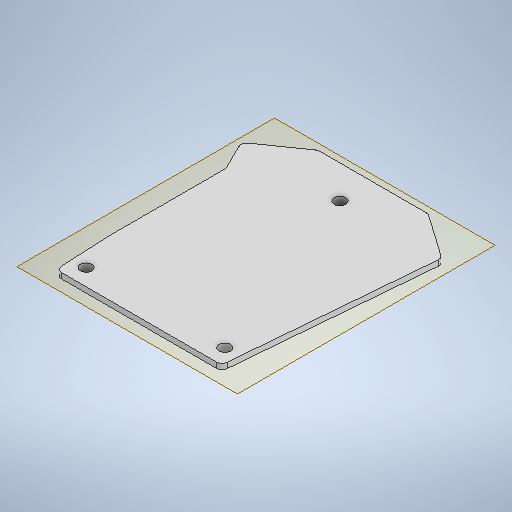
# Autodesk Inventor part: Deckel_oberteil
Saved by Autodesk Inventor 2025.1 (Build 291241000, 241)
## iProperties
Created: 2025-02-01
Part Number: Deckel_oberteil
Material: Generisch
Document SubType Name: Modeling
Designer: joebe
Density: 1 g/cm^3
Appearance: Vorgabe
Author: joebe
Autodesk Inventor part; units mm, degrees
ref_plane "YZ Plane" through (0, 0, 0) normal (1, 0, 0) x (0, 1, 0)
ref_plane "XZ Plane" through (0, 0, 0) normal (0, 1, 0) x (-1, 0, 0)
ref_plane "XY Plane" through (0, 0, 0) normal (0, 0, 1) x (1, 0, 0)
ref_plane "Arbeitsebene1" through (0, 0, 0) normal (0, 0, 1) x (1, 0, 0)
sketch "Skizze1" plane through (0, 0, 0) normal (0, 0, 1) x (1, 0, 0)
  line L0 (-29, -22.45) -> (-29, 20.1) projected
  line L1 (-29.2058, 20.9837) -> (-32.4027, 27.4738) projected
  line L2 (-17.2708, 40.1383) -> (-31.7557, 29.9959) projected
  line L3 (-16.1236, 40.5) -> (16.1236, 40.5) projected
  line L4 (33.1958, 28.9875) -> (17.2708, 40.1383) projected
  line L5 (34.0411, 27.1762) -> (28.1661, -40.5) projected
  line L6 (28.1661, -40.5) -> (-28.0975, -40.5) projected
  line L7 (-28.0975, -40.5) -> (-29, -22.45) projected
  line L8 (-30.9975, -22.5499) -> (-30.095, -40.5999) projected
  line L9 (-28.0975, -42.5) -> (28.1661, -42.5) projected
  line L10 (30.1586, -40.673) -> (36.2833, 29.879) projected
  line L11 (35.4379, 31.6903) -> (20.5166, 42.1383) projected
  line L12 (19.3694, 42.5) -> (-19.3694, 42.5) projected
  line L13 (-20.5166, 42.1383) -> (-34.9783, 32.0121) projected
  line L14 (-35.6253, 29.4901) -> (-31.2058, 20.5179) projected
  line L15 (-31, 19.6342) -> (-31, -22.45) projected
  line L16 (-32.5225, 28.8486) -> (-28.5, 20.6823)
  line L17 (-28.5, 20.6823) -> (-28.5, -22.4375)
  line L18 (-28.5, -22.4375) -> (-27.6219, -40)
  line L19 (-27.6219, -40) -> (27.7076, -40)
  line L20 (27.7076, -40) -> (33.6178, 28.0816)
  line L21 (33.6178, 28.0816) -> (16.5966, 40)
  line L22 (16.5966, 40) -> (-16.5966, 40)
  line L23 (-16.5966, 40) -> (-32.5225, 28.8486)
  arc A0 (-29, 20.1) -> (-29.2058, 20.9837) centre (-31, 20.1) ccw projected
  arc A1 (-31.7557, 29.9959) -> (-32.4027, 27.4738) centre (-30.6085, 28.3576) ccw projected
  arc A2 (-16.1236, 40.5) -> (-17.2708, 40.1383) centre (-16.1236, 38.5) ccw projected
  arc A3 (17.2708, 40.1383) -> (16.1236, 40.5) centre (16.1236, 38.5) ccw projected
  arc A4 (34.0411, 27.1762) -> (33.1958, 28.9875) centre (32.0486, 27.3492) ccw projected
  arc A5 (-31, -22.45) -> (-30.9975, -22.5499) centre (-29, -22.45) ccw projected
  arc A6 (-30.095, -40.5999) -> (-28.0975, -42.5) centre (-28.0975, -40.5) ccw projected
  arc A7 (28.1661, -42.5) -> (30.1586, -40.673) centre (28.1661, -40.5) ccw projected
  arc A8 (36.2833, 29.879) -> (35.4379, 31.6903) centre (34.2907, 30.052) ccw projected
  arc A9 (20.5166, 42.1383) -> (19.3694, 42.5) centre (19.3694, 40.5) ccw projected
  arc A10 (-19.3694, 42.5) -> (-20.5166, 42.1383) centre (-19.3694, 40.5) ccw projected
  arc A11 (-34.9783, 32.0121) -> (-35.6253, 29.4901) centre (-33.8311, 30.3738) ccw projected
  arc A12 (-31, 19.6342) -> (-31.2058, 20.5179) centre (-33, 19.6342) ccw projected
  point P0 (0, 0)
  dimension "d2" = 0.5
  constraints: 16 end point, 7 other
  measures "d2" distance between parallel lines of L2 L23
extrude "Extrusion1" add sketch "Skizze1" against normal blind 2 contours L23 L22 L21 L20 L19 L18 L17 L16
sketch "Skizze2" plane through (0, 0, 0) normal (0, 0, 1) x (-1, 0, 0)
  point P0 (0, 0)
sketch "Skizze3" plane through (0, 0, 0) normal (0, 0, 1) x (1, 0, 0)
  line L0 (-29, -22.45) -> (-29, 20.1) projected
  line L1 (-29.2058, 20.9837) -> (-32.4027, 27.4738) projected
  line L2 (-17.2708, 40.1383) -> (-31.7557, 29.9959) projected
  line L3 (-16.1236, 40.5) -> (16.1236, 40.5) projected
  line L4 (33.1958, 28.9875) -> (17.2708, 40.1383) projected
  line L5 (34.0411, 27.1762) -> (28.1661, -40.5) projected
  line L6 (28.1661, -40.5) -> (-28.0975, -40.5) projected
  line L7 (-28.0975, -40.5) -> (-29, -22.45) projected
  line L8 (-30.9975, -22.5499) -> (-30.095, -40.5999) projected
  line L9 (-28.0975, -42.5) -> (28.1661, -42.5) projected
  line L10 (30.1586, -40.673) -> (36.2833, 29.879) projected
  line L11 (35.4379, 31.6903) -> (20.5166, 42.1383) projected
  line L12 (19.3694, 42.5) -> (-19.3694, 42.5) projected
  line L13 (-20.5166, 42.1383) -> (-34.9783, 32.0121) projected
  line L14 (-35.6253, 29.4901) -> (-31.2058, 20.5179) projected
  line L15 (-31, 19.6342) -> (-31, -22.45) projected
  arc A0 (-29, 20.1) -> (-29.2058, 20.9837) centre (-31, 20.1) ccw projected
  arc A1 (-31.7557, 29.9959) -> (-32.4027, 27.4738) centre (-30.6085, 28.3576) ccw projected
  arc A2 (-16.1236, 40.5) -> (-17.2708, 40.1383) centre (-16.1236, 38.5) ccw projected
  arc A3 (17.2708, 40.1383) -> (16.1236, 40.5) centre (16.1236, 38.5) ccw projected
  arc A4 (34.0411, 27.1762) -> (33.1958, 28.9875) centre (32.0486, 27.3492) ccw projected
  arc A5 (-31, -22.45) -> (-30.9975, -22.5499) centre (-29, -22.45) ccw projected
  arc A6 (-30.095, -40.5999) -> (-28.0975, -42.5) centre (-28.0975, -40.5) ccw projected
  arc A7 (28.1661, -42.5) -> (30.1586, -40.673) centre (28.1661, -40.5) ccw projected
  arc A8 (36.2833, 29.879) -> (35.4379, 31.6903) centre (34.2907, 30.052) ccw projected
  arc A9 (20.5166, 42.1383) -> (19.3694, 42.5) centre (19.3694, 40.5) ccw projected
  arc A10 (-19.3694, 42.5) -> (-20.5166, 42.1383) centre (-19.3694, 40.5) ccw projected
  arc A11 (-34.9783, 32.0121) -> (-35.6253, 29.4901) centre (-33.8311, 30.3738) ccw projected
  arc A12 (-31, 19.6342) -> (-31.2058, 20.5179) centre (-33, 19.6342) ccw projected
  point P0 (0, 0)
extrude "Extrusion2" add sketch "Skizze3" along normal blind 2 contours L0 A0 L1 A1 L2 A2 L3 A3 L4 A4 L5 L6 L7 | A5 L15 A12 L14 A11 L13 A10 L12 A9 L11 A8 L10 A7 L9 A6 L8
sketch "Skizze4" plane through (0, 0, 2) normal (0, 0, 1) x (1, 0, 0)
  circle A0 centre (-25.2, -36.5) radius 1.5 projected
  circle A1 centre (25.2, -36.5) radius 1.5 projected
  circle A2 centre (0, 30.5) radius 1.5 projected
  point P0 (0, 0)
hole "Bohrung1" at (0, 30.5, 2) at (25.2, -36.5, 2) at (-25.2, -36.5, 2) direction (0, 0, -1) diameter 4.2 end through all
fillet "Rundung1" radius 2 6 edges at (27.7076, -40, -1) (-27.6219, -40, -1) (33.6178, 28.0816, -1) (16.5966, 40, -1) (-32.5225, 28.8486, -1) (-16.5966, 40, -1)
